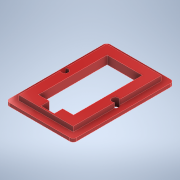
# Autodesk Inventor part: servo_cover2
Saved by Autodesk Inventor 2022 (Build 260153000, 153)
## iProperties
Created: 2024-10-10
Part Number: servo_cover2
Material: 一般
Document SubType Name: Modeling
Designer: rugby
Density: 1 g/cm^3
Appearance: 赤
Author: rugby
## iProperties of the stored document servo_cover2_3D プリント.ipt
Created: 2024-10-20
Part Number: servo_cover2_3D プリント
Material: 一般
Document SubType Name: Modeling
Designer: acbaf
Density: 1 g/cm^3
Appearance: 既定
Author: acbaf
Autodesk Inventor part; units mm, degrees
ref_plane "YZ Plane" through (0, 0, 0) normal (1, 0, 0) x (0, 1, 0)
ref_plane "XZ Plane" through (0, 0, 0) normal (0, 1, 0) x (-1, 0, 0)
ref_plane "XY Plane" through (0, 0, 0) normal (0, 0, 1) x (1, 0, 0)
sketch "スケッチ1" plane through (0, 0, 0) normal (0, 1, 0) x (-1, 0, 0)
  circle A0 centre (15, 44.75) radius 2
  circle A1 centre (5, 44.75) radius 2
  circle A2 centre (10, 30) radius 3
  circle A3 centre (15, -4.75) radius 2
  circle A4 centre (5, -4.75) radius 2
  circle A5 centre (10, 30) radius 3
  line L0 (0, 0) -> (0, 40)
  line L1 (20, 0) -> (0, 0)
  line L2 (20, 40) -> (20, 0)
  line L3 (0, 40) -> (20, 40)
  line L4 (0, 40) -> (20, 40)
  line L5 (20, 45.25) -> (20, 40)
  arc A6 (20, 45.25) -> (18, 47.447) centre (18.0097, 45.4471) ccw
  line L6 (2, 47.447) -> (18, 47.447)
  arc A7 (2, 47.447) -> (0, 45.25) centre (1.9903, 45.4471) ccw
  line L7 (0, 40) -> (0, 45.25)
  circle A8 centre (15, 44.75) radius 2
  circle A9 centre (5, 44.75) radius 2
  line L8 (20, 0) -> (0, 0)
  line L9 (0, -5.25) -> (0, 0)
  arc A10 (0, -5.25) -> (2, -7.25) centre (2, -5.25) ccw
  line L10 (18, -7.25) -> (2, -7.25)
  arc A11 (18, -7.25) -> (20, -5.25) centre (18, -5.25) ccw
  line L11 (20, 0) -> (20, -5.25)
  circle A12 centre (5, -4.75) radius 2
  circle A13 centre (15, -4.75) radius 2
  line L12 (-8, 50.197) -> (28, 50.197)
  line L13 (30, 48.197) -> (30, -7.803)
  line L14 (28, -9.803) -> (-8, -9.803)
  line L15 (-10, -7.803) -> (-10, 48.197)
  arc A14 (30, 48.197) -> (28, 50.197) centre (28, 48.197) ccw
  arc A15 (-8, 50.197) -> (-10, 48.197) centre (-8, 48.197) ccw
  arc A16 (-10, -7.803) -> (-8, -9.803) centre (-8, -7.803) ccw
  arc A17 (28, -9.803) -> (30, -7.803) centre (28, -7.803) ccw
  line L16 (45.2724, 20.197) -> (-29.952, 20.197)
  line L17 (25, 53.3822) -> (25, -21.2286)
  line L18 (-5, 50.197) -> (-5, -9.803)
  line L19 (6.5, 45) -> (13.5, 45)
  line L20 (13.5, 45) -> (13.5, 40)
  line L21 (6.5, 40) -> (6.5, 45)
  line L22 (0, 40) -> (20, 40)
  point P0 (0, -4.75)
  point P1 (-10, 50.197)
  point P2 (30, -9.803)
  point P3 (30, 50.197)
  point P4 (10, 47.447)
  point P5 (10, 50.197)
  point P6 (-5, 20.197)
  point P7 (-5, 20.197)
  point P8 (25, 20.197)
  point P9 (25, 50.197)
  point P10 (25, -9.803)
  dimension "d0" = 40
  dimension "d1" = 60
  dimension "d2" = 2.75
  dimension "d3" = 10
  dimension "d4" = 2
  dimension "d5" = 30
  dimension "d6" = 5
  dimension "d7" = 5
  dimension "d8" = 60
  dimension "d9" = 0
  dimension "d22" = 2.75
  dimension "d23" = 2
  dimension "d24" = 2
  dimension "d25" = 10
  dimension "d26" = 15
  dimension "d27" = 5.447
  dimension "d28" = 10
  dimension "d29" = 20
  dimension "d30" = 20.197
  constraints: 46 end point, 18 centre point, 16 point on circle, 9 point on line, 8 tangent, 4 midpoint, 3 equal radius, 3 parallel, 2 horizontal, 1 perpendicular, 1 vertical
  measures "d0" distance of point (-10, 50.197) point (30, 50.197)
  measures "d1" distance of point (30, 50.197) point (30, -9.803)
  measures "d2" distance of point (10, 47.447) point (10, 50.197)
  measures "d3" distance between parallel lines of L13 L2
  measures "d4" radius of A14
  measures "d5" distance between parallel lines of L14 L16
  measures "d6" distance between parallel lines of L17 L13
  measures "d7" distance from line of L15 point (-5, 20.197)
  measures "d8" distance of L18.start L18.end
  measures "d9" distance from line of L18.start L12
  measures "d22" distance from line of L6.end L12
  measures "d23" radius of A6
  measures "d24" radius of A7
  measures "d25" distance of A0.centre A1.centre
  measures "d26" distance from line of L13 A0.centre
  measures "d27" distance from line of L12 A0.centre
  measures "d28" distance from line of A2.centre L3
  measures "d29" distance from line of L15 A2.centre
  measures "d30" distance from line of A2.centre L12
extrude "押し出し1" add sketch "スケッチ1" along normal blind 5 contours A0 L20 L19 | A0 L19 A1 L21 L3 L7 A7 L6 A6 L5 L20 | L19 L21 A1 | L5 A6 L6 A7 L7 L0 L16 L18 L12 L17 L2 | L16 L17 L14 L18 L0 L9 A10 L10 A11 L11 L2 | L11 A11 L10 A10 L9 L1 | L17 L12 A14 L13 L16 | L16 L13 A17 L14 L17 | L18 L14 A16 L15 L16 | L16 L15 A15 L12 L18 | A3 | A4 picked at (15.8139, 44.6736) picked at (4.1802, 44.7383)
hole "穴1" at (5, 0, 20.197) at (-25, 0, 20.197) direction (0, 1, 0) diameter 4 end through all
sketch "スケッチ2" plane through (0, 5, 0) normal (0, 1, 0) x (1, 0, 0)
  circle A0 centre (5, -20.197) radius 2 projected
  circle A1 centre (-25, -20.197) radius 2 projected
  line L0 (-28, -50.197) -> (8, -50.197) projected
  arc A2 (8, -50.197) -> (10, -48.197) centre (8, -48.197) ccw projected
  line L1 (10, -48.197) -> (10, 7.803) projected
  arc A3 (10, 7.803) -> (8, 9.803) centre (8, 7.803) ccw projected
  line L2 (8, 9.803) -> (-28, 9.803) projected
  arc A4 (-28, 9.803) -> (-30, 7.803) centre (-28, 7.803) ccw projected
  line L3 (-30, 7.803) -> (-30, -48.197) projected
  arc A5 (-30, -48.197) -> (-28, -50.197) centre (-28, -48.197) ccw projected
  line L4 (-20, -40) -> (-20, 0) projected
  line L5 (-20, 0) -> (0, 0) projected
  line L6 (0, 0) -> (0, -40) projected
  line L7 (0, -40) -> (-6.5, -40) projected
  line L8 (-6.5, -40) -> (-6.5, -45) projected
  line L9 (-6.5, -45) -> (-13.5, -45) projected
  line L10 (-13.5, -45) -> (-13.5, -40) projected
  line L11 (-13.5, -40) -> (-20, -40) projected
  line L12 (-6, -40.5) -> (0.5, -40.5)
  line L13 (0.5, -40.5) -> (0.5, 0.5)
  line L14 (0.5, 0.5) -> (-20.5, 0.5)
  line L15 (-20.5, 0.5) -> (-20.5, -40.5)
  line L16 (-20.5, -40.5) -> (-14, -40.5)
  line L17 (-14, -40.5) -> (-14, -45.5)
  line L18 (-14, -45.5) -> (-6, -45.5)
  line L19 (-6, -45.5) -> (-6, -40.5)
  dimension "d19" = 0.5
  constraints: 16 end point, 7 other
  measures "d19" distance between parallel lines of L7 L12
extrude "押し出し2" cut sketch "スケッチ2" against normal blind 10 contours L19 L18 L17 L16 L15 L14 L13 L12
sketch "スケッチ3" plane through (0, 5, 0) normal (0, 1, 0) x (1, 0, 0)
  line L0 (10, -48.197) -> (10, 7.803) projected
  arc A0 (8, -50.197) -> (10, -48.197) centre (8, -48.197) ccw projected
  line L1 (-28, -50.197) -> (8, -50.197) projected
  arc A1 (-30, -48.197) -> (-28, -50.197) centre (-28, -48.197) ccw projected
  line L2 (-30, 7.803) -> (-30, -48.197) projected
  arc A2 (-28, 9.803) -> (-30, 7.803) centre (-28, 7.803) ccw projected
  line L3 (8, 9.803) -> (-28, 9.803) projected
  arc A3 (10, 7.803) -> (8, 9.803) centre (8, 7.803) ccw projected
  line L4 (6.2, -46.397) -> (6.2, 6.003)
  line L5 (6.2, 6.003) -> (-26.2, 6.003)
  line L6 (-26.2, 6.003) -> (-26.2, -46.397)
  line L7 (-26.2, -46.397) -> (6.2, -46.397)
  point P0 (0, 0)
  dimension "d31" = 3.8
  constraints: 8 end point, 3 other
  measures "d31" distance between parallel lines of L1 L7
extrude "押し出し3" cut sketch "スケッチ3" against normal blind 3
equation "\"d5\" = 0.5 * d1"
equation "\"d6\" = 0.5 * d3"
equation "\"d7\" = d6"
equation "\"d8\" = d1"
